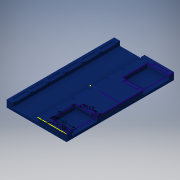
# Autodesk Inventor part: Assembly Plate
Saved by Autodesk Inventor 2019.4 (Build 234330000, 330)
## iProperties
Created: 2021-01-11
Part Number: Assembly Plate
Material: Aluminum, Anodized Blue
Document SubType Name: Modeling
Designer: caleb
Density: 2.7 g/cm^3
Appearance: Anodized - Blue
Author: caleb
Autodesk Inventor part; units mm, degrees
ref_plane "YZ Plane" through (0, 0, 0) normal (1, 0, 0) x (0, 1, 0)
ref_plane "XZ Plane" through (0, 0, 0) normal (0, 1, 0) x (-1, 0, 0)
ref_plane "XY Plane" through (0, 0, 0) normal (0, 0, 1) x (1, 0, 0)
sketch "Sketch1" plane through (0, 0, 0) normal (0, 1, 0) x (-1, 0, 0)
  line L0 (-60, 108) -> (60, 108)
  line L1 (60, 108) -> (60, -108)
  line L2 (60, -108) -> (-60, -108)
  line L3 (-60, -108) -> (-60, 108)
  line L4 (-60, 108) -> (60, -108) construction
  line L5 (60, 108) -> (-60, -108) construction
  point P0 (0, 0)
  dimension "d0" = 120
  dimension "d1" = 216
  constraints: 12 end point, 2 midpoint, 2 parallel, 1 horizontal, 1 perpendicular
  measures "d0" distance of L1.end L2.end
  measures "d1" distance of L0.end L1.end
extrude "Extrusion1" add sketch "Sketch1" along normal blind 14
sketch "Sketch8" plane through (0, 14, 0) normal (0, 1, 0) x (1, 0, 0)
  line L0 (-60, -108) -> (60, -108) projected
  line L1 (60, 108) -> (-60, 108) projected
  line L2 (-60, 108) -> (-60, -108) projected
  line L3 (60, -108) -> (60, 108) projected
  line L4 (-49, -108) -> (1, -108)
  line L5 (1, -108) -> (1, 108)
  line L6 (1, 108) -> (-49, 108)
  line L7 (-49, 108) -> (-49, -108)
  point P0 (0, 0)
  dimension "d91" = 11
  dimension "d92" = 50
  constraints: 8 end point, 2 parallel, 2 point on line, 1 horizontal, 1 perpendicular
  measures "d91" distance between parallel lines of L2 L7
  measures "d92" distance between parallel lines of L7 L5
extrude "Extrusion7" cut sketch "Sketch8" against normal blind 9 contours L7 L1 L5 L0
sketch "Sketch9" plane through (0, 14, 0) normal (0, 1, 0) x (1, 0, 0)
  line L0 (-60, -108) -> (-49, -108) projected
  line L1 (-60, 108) -> (-60, -108) projected
  line L2 (-49, -108) -> (-49, 108) projected
  line L3 (-49, -100.972) -> (-55.5, -100.972)
  line L4 (-55.5, -100.972) -> (-55.5, -74.172)
  line L5 (-54.5, -73.172) -> (-49, -73.172)
  line L6 (-49, -73.172) -> (-49, -100.972)
  circle A0 centre (-55.5, -100.972) radius 1
  line L7 (1, 108) -> (1, -108) projected
  line L8 (1, -108) -> (60, -108) projected
  line L9 (1, -100.972) -> (6.5, -100.972)
  line L10 (7.5, -99.972) -> (7.5, -74.172)
  line L11 (6.5, -73.172) -> (1, -73.172)
  line L12 (1, -73.172) -> (1, -100.972)
  arc A1 (-54.5, -73.172) -> (-55.5, -74.172) centre (-54.5, -74.172) ccw
  arc A2 (7.5, -74.172) -> (6.5, -73.172) centre (6.5, -74.172) ccw
  arc A3 (6.5, -100.972) -> (7.5, -99.972) centre (6.5, -99.972) ccw
  arc A4 (7.5, -39.344) -> (6.5, -38.344) centre (6.5, -39.344) ccw
  line L13 (1, -38.344) -> (1, -66.144)
  line L14 (7.5, -65.144) -> (7.5, -39.344)
  line L15 (1, -66.144) -> (6.5, -66.144)
  arc A5 (6.5, -66.144) -> (7.5, -65.144) centre (6.5, -65.144) ccw
  line L16 (6.5, -38.344) -> (1, -38.344)
  line L17 (-49, -38.344) -> (-49, -66.144)
  line L18 (-54.5, -38.344) -> (-49, -38.344)
  arc A6 (-54.5, -38.344) -> (-55.5, -39.344) centre (-54.5, -39.344) ccw
  line L19 (-55.5, -66.144) -> (-55.5, -39.344)
  line L20 (-49, -66.144) -> (-55.5, -66.144)
  circle A7 centre (-55.5, -66.144) radius 1
  arc A8 (7.5, -4.516) -> (6.5, -3.516) centre (6.5, -4.516) ccw
  line L21 (1, -3.516) -> (1, -31.316)
  line L22 (7.5, -30.316) -> (7.5, -4.516)
  line L23 (1, -31.316) -> (6.5, -31.316)
  arc A9 (6.5, -31.316) -> (7.5, -30.316) centre (6.5, -30.316) ccw
  line L24 (6.5, -3.516) -> (1, -3.516)
  line L25 (-49, -3.516) -> (-49, -31.316)
  line L26 (-54.5, -3.516) -> (-49, -3.516)
  arc A10 (-54.5, -3.516) -> (-55.5, -4.516) centre (-54.5, -4.516) ccw
  line L27 (-55.5, -31.316) -> (-55.5, -4.516)
  line L28 (-49, -31.316) -> (-55.5, -31.316)
  circle A11 centre (-55.5, -31.316) radius 1
  arc A12 (7.5, 30.312) -> (6.5, 31.312) centre (6.5, 30.312) ccw
  line L29 (1, 31.312) -> (1, 3.512)
  line L30 (7.5, 4.512) -> (7.5, 30.312)
  line L31 (1, 3.512) -> (6.5, 3.512)
  arc A13 (6.5, 3.512) -> (7.5, 4.512) centre (6.5, 4.512) ccw
  line L32 (6.5, 31.312) -> (1, 31.312)
  line L33 (-49, 31.312) -> (-49, 3.512)
  line L34 (-54.5, 31.312) -> (-49, 31.312)
  arc A14 (-54.5, 31.312) -> (-55.5, 30.312) centre (-54.5, 30.312) ccw
  line L35 (-55.5, 3.512) -> (-55.5, 30.312)
  line L36 (-49, 3.512) -> (-55.5, 3.512)
  circle A15 centre (-55.5, 3.512) radius 1
  arc A16 (7.5, 65.14) -> (6.5, 66.14) centre (6.5, 65.14) ccw
  line L37 (1, 66.14) -> (1, 38.34)
  line L38 (7.5, 39.34) -> (7.5, 65.14)
  line L39 (1, 38.34) -> (6.5, 38.34)
  arc A17 (6.5, 38.34) -> (7.5, 39.34) centre (6.5, 39.34) ccw
  line L40 (6.5, 66.14) -> (1, 66.14)
  line L41 (-49, 66.14) -> (-49, 38.34)
  line L42 (-54.5, 66.14) -> (-49, 66.14)
  arc A18 (-54.5, 66.14) -> (-55.5, 65.14) centre (-54.5, 65.14) ccw
  line L43 (-55.5, 38.34) -> (-55.5, 65.14)
  line L44 (-49, 38.34) -> (-55.5, 38.34)
  circle A19 centre (-55.5, 38.34) radius 1
  arc A20 (7.5, 99.968) -> (6.5, 100.968) centre (6.5, 99.968) ccw
  line L45 (1, 100.968) -> (1, 73.168)
  line L46 (7.5, 74.168) -> (7.5, 99.968)
  line L47 (1, 73.168) -> (6.5, 73.168)
  arc A21 (6.5, 73.168) -> (7.5, 74.168) centre (6.5, 74.168) ccw
  line L48 (6.5, 100.968) -> (1, 100.968)
  line L49 (-49, 100.968) -> (-49, 73.168)
  line L50 (-54.5, 100.968) -> (-49, 100.968)
  arc A22 (-54.5, 100.968) -> (-55.5, 99.968) centre (-54.5, 99.968) ccw
  line L51 (-55.5, 73.168) -> (-55.5, 99.968)
  line L52 (-49, 73.168) -> (-55.5, 73.168)
  circle A23 centre (-55.5, 73.168) radius 1
  point P0 (0, 0)
  point P1 (-55.5, -73.172)
  point P2 (7.5, -73.172)
  point P3 (7.5, -100.972)
  point P4 (7.5, -38.344)
  point P5 (7.5, -66.144)
  point P6 (-55.5, -38.344)
  point P7 (7.5, -3.516)
  point P8 (7.5, -31.316)
  point P9 (-55.5, -3.516)
  point P10 (7.5, 31.312)
  point P11 (7.5, 3.512)
  point P12 (-55.5, 31.312)
  point P13 (7.5, 66.14)
  point P14 (7.5, 38.34)
  point P15 (-55.5, 66.14)
  point P16 (7.5, 100.968)
  point P17 (7.5, 73.168)
  point P18 (-55.5, 100.968)
  dimension "d95" = 7.028
  dimension "d96" = 27.8
  dimension "d97" = 2
  dimension "d99" = 6.5
  dimension "d100" = 7.028
  dimension "d101" = 27.8
  dimension "d102" = 6.5
  dimension "d105" = 1
  dimension "d108" = 34.828
  constraints: 96 end point, 38 point on line, 36 point on circle, 24 centre point, 6 coincident, 6 tangent, 4 parallel, 2 equal radius, 2 horizontal, 2 perpendicular, 1 vertical, 150 other
  measures "d95" distance between parallel lines of L0 L3
  measures "d96" distance of L3.end point (-55.5, -73.172)
  measures "d97" diameter of A0
  measures "d99" distance of L3.start L3.end
  measures "d100" distance between parallel lines of L8 L9
  measures "d101" distance of point (7.5, -100.972) point (7.5, -73.172)
  measures "d102" distance of point (7.5, -73.172) L11.end
  measures "d105" radius of A1
  measures "d108" distance of L11.end L13.start
extrude "Extrusion8" cut sketch "Sketch9" against normal blind 2
sketch "Sketch10" plane through (0, 14, 0) normal (0, 1, 0) x (1, 0, 0)
  line L0 (60, 108) -> (60, -108) projected
  line L1 (60, -97) -> (19, -97)
  line L2 (18, -96) -> (18, -48)
  line L3 (19, -47) -> (60, -47)
  line L4 (60, -47) -> (60, -97)
  line L5 (1, -108) -> (60, -108) projected
  line L6 (52.972, -97) -> (25.172, -97)
  line L7 (25.172, -97) -> (25.172, -102.5)
  line L8 (26.172, -103.5) -> (52.972, -103.5)
  line L9 (52.972, -103.5) -> (52.972, -97)
  line L10 (52.972, -47) -> (25.172, -47)
  line L11 (25.172, -47) -> (25.172, -41.5)
  line L12 (26.172, -40.5) -> (51.972, -40.5)
  line L13 (52.972, -41.5) -> (52.972, -47)
  circle A0 centre (52.972, -103.5) radius 1
  arc A1 (25.172, -102.5) -> (26.172, -103.5) centre (26.172, -102.5) ccw
  arc A2 (26.172, -40.5) -> (25.172, -41.5) centre (26.172, -41.5) ccw
  arc A3 (52.972, -41.5) -> (51.972, -40.5) centre (51.972, -41.5) ccw
  arc A4 (19, -47) -> (18, -48) centre (19, -48) ccw
  arc A5 (18, -96) -> (19, -97) centre (19, -96) ccw
  line L14 (60, 0) -> (16.2003, 0)
  line L15 (60, -108) -> (60, 108)
  line L16 (60, 97) -> (19, 97)
  line L17 (18, 96) -> (18, 48)
  line L18 (19, 47) -> (60, 47)
  line L19 (60, 47) -> (60, 97)
  line L20 (52.972, 97) -> (25.172, 97)
  line L21 (25.172, 97) -> (25.172, 102.5)
  line L22 (26.172, 103.5) -> (52.972, 103.5)
  line L23 (52.972, 103.5) -> (52.972, 97)
  line L24 (52.972, 47) -> (25.172, 47)
  line L25 (25.172, 47) -> (25.172, 41.5)
  line L26 (26.172, 40.5) -> (51.972, 40.5)
  line L27 (52.972, 41.5) -> (52.972, 47)
  circle A6 centre (52.972, 103.5) radius 1
  arc A7 (26.172, 103.5) -> (25.172, 102.5) centre (26.172, 102.5) ccw
  arc A8 (25.172, 41.5) -> (26.172, 40.5) centre (26.172, 41.5) ccw
  arc A9 (51.972, 40.5) -> (52.972, 41.5) centre (51.972, 41.5) ccw
  arc A10 (18, 48) -> (19, 47) centre (19, 48) ccw
  arc A11 (19, 97) -> (18, 96) centre (19, 96) ccw
  point P0 (0, 0)
  point P1 (18, -47)
  point P2 (18, -97)
  point P3 (25.172, -103.5)
  point P4 (25.172, -40.5)
  point P5 (52.972, -40.5)
  point P6 (18, 47)
  point P7 (18, 97)
  point P8 (25.172, 103.5)
  point P9 (25.172, 40.5)
  point P10 (52.972, 40.5)
  dimension "d115" = 50
  dimension "d116" = 11
  dimension "d117" = 42
  dimension "d118" = 7.028
  dimension "d119" = 27.8
  dimension "d120" = 6.5
  dimension "d121" = 6.5
  dimension "d122" = 7.028
  dimension "d123" = 27.8
  dimension "d124" = 2
  dimension "d125" = 1
  constraints: 52 end point, 30 symmetric about line, 26 point on line, 20 point on circle, 12 centre point, 10 tangent, 6 parallel, 4 equal radius, 4 horizontal, 3 perpendicular, 2 coincident, 1 midpoint, 6 other
  measures "d115" distance of point (18, -97) point (18, -47)
  measures "d116" distance between parallel lines of L5 L1
  measures "d117" distance of L1.start point (18, -97)
  measures "d118" distance between parallel lines of L0 L9
  measures "d119" distance of point (25.172, -103.5) L8.end
  measures "d120" distance between parallel lines of L8 L6
  measures "d121" distance of L10.end point (25.172, -40.5)
  measures "d122" distance between parallel lines of L0 L13
  measures "d123" distance of point (25.172, -40.5) point (52.972, -40.5)
  measures "d124" diameter of A0
  measures "d125" radius of A1
extrude "Extrusion9" cut sketch "Sketch10" against normal blind 9 contours L0 L18 A10 L17 A11 L16 | L0 L1 A5 L2 A4 L3
extrude "Extrusion10" cut sketch "Sketch10" against normal blind 2 contours L16 L21 A7 L22 A6 L23 | L27 A9 L26 A8 L25 L18 | A6 L22 L23 | L23 L22 A6 | L3 L11 A2 L12 A3 L13 | L9 A0 L8 A1 L7 L1 | A0 L8 L9 | L9 L8 A0
body "Solid1"
